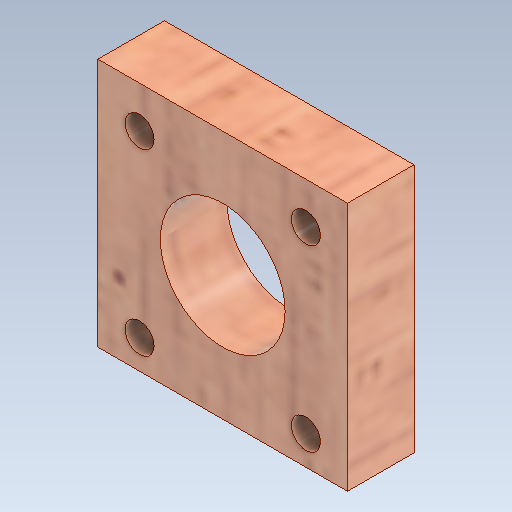
# Autodesk Inventor part: 0005-10-006 Capac rulment
Saved by Autodesk Inventor 2020 (Build 240168000, 168)
## iProperties
Created: 2020-12-18
Part Number: 0005-10-006 Capac rulment
Material: Generic
Document SubType Name: Modeling
Designer: Iulian Bors
Density: 1 g/cm^3
Appearance: White Oak - Natural Medium Gloss
Author: Iulian Bors
Subject: 006
Autodesk Inventor part; units mm, degrees
ref_plane "YZ Plane" through (0, 0, 0) normal (1, 0, 0) x (0, 1, 0)
ref_plane "XZ Plane" through (0, 0, 0) normal (0, 1, 0) x (-1, 0, 0)
ref_plane "XY Plane" through (0, 0, 0) normal (0, 0, 1) x (1, 0, 0)
sketch "Sketch1" plane through (0, 0, 0) normal (0, 0, 1) x (1, 0, 0)
  line L0 (-15, 15) -> (15, 15)
  line L1 (15, 15) -> (15, -15)
  line L2 (15, -15) -> (-15, -15)
  line L3 (-15, -15) -> (-15, 15)
  point P0 (0, 0)
  point P1 (0, 15)
  point P2 (-15, 0)
  dimension "d0" = 30
  dimension "d1" = 30
  constraints: 8 end point, 2 midpoint, 2 parallel, 1 horizontal, 1 horizontal alignment, 1 perpendicular, 1 vertical alignment
  measures "d0" distance of L0.start L0.end
  measures "d1" distance of L2.end L0.start
extrude "Extrusion1" add sketch "Sketch1" along normal blind 8
sketch "Sketch2" plane through (0, 0, 8) normal (0, 0, 1) x (1, 0, 0)
  circle A0 centre (0, 0) radius 7.5
  line L0 (15, 15) -> (-15, 15) projected
  line L1 (-15, 15) -> (-15, -15) projected
  point P0 (0, 15)
  point P1 (-15, 0)
  dimension "d17" = 15
  constraints: 2 midpoint, 1 centre point, 1 horizontal alignment, 1 vertical alignment
  measures "d17" diameter of A0
extrude "Extrusion2" cut sketch "Sketch2" against normal through all
sketch "Sketch3" plane through (0, 0, 8) normal (0, 0, 1) x (1, 0, 0)
  circle A0 centre (10, -11.5) radius 1.75
  circle A1 centre (10, 10) radius 1.75
  line L0 (15, 15) -> (-15, 15) projected
  line L1 (15, -15) -> (15, 15) projected
  circle A2 centre (-10, -11.5) radius 1.75
  circle A3 centre (-10, 10) radius 1.75
  line L2 (-15, 15) -> (-15, -15) projected
  line L3 (-15, -15) -> (15, -15) projected
  point P0 (0, 0)
  dimension "d9" = 3.5
  dimension "d10" = 3.5
  dimension "d12" = 5
  dimension "d13" = 5
  dimension "d14" = 5
  dimension "d18" = 3.5
  constraints: 4 centre point, 2 equal radius, 2 horizontal alignment, 2 vertical alignment
  measures "d9" diameter of A0
  measures "d10" diameter of A1
  measures "d12" distance from line of A1.centre L0
  measures "d13" distance from line of L1 A0.centre
  measures "d14" distance from line of A2.centre L2
  measures "d18" distance from line of L3 A0.centre
extrude "Extrusion3" cut sketch "Sketch3" against normal through all contours A0 | A1 | A2 | A3
equation "\"d14\" = d13"
body "Solid1"
